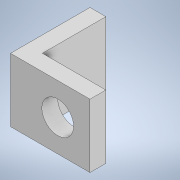
# Autodesk Inventor part: sideSupport
Saved by Autodesk Inventor 2022.2 (Build 262287010, 287A)
## iProperties
Created: 2022-09-12
Part Number: sideSupport
Material: Generic
Document SubType Name: Modeling
Designer: robst
Density: 1 g/cm^3
Appearance: Default
Author: robst
Autodesk Inventor part; units mm, degrees
ref_plane "YZ Plane" through (0, 0, 0) normal (1, 0, 0) x (0, 1, 0)
ref_plane "XZ Plane" through (0, 0, 0) normal (0, 1, 0) x (-1, 0, 0)
ref_plane "XY Plane" through (0, 0, 0) normal (0, 0, 1) x (1, 0, 0)
sketch "Sketch1" plane through (0, 0, 0) normal (1, 0, 0) x (0, 1, 0)
  line L0 (-12.7, 15.875) -> (-12.7, -15.875)
  line L1 (-12.7, -15.875) -> (12.7, -15.875)
  line L2 (12.7, -15.875) -> (12.7, 15.875)
  line L3 (12.7, 15.875) -> (-12.7, 15.875)
  line L4 (-12.7, 15.875) -> (12.7, -15.875) construction
  line L5 (-12.7, -15.875) -> (12.7, 15.875) construction
  point P0 (0, 0)
  dimension "d0" = 25.4
  dimension "d1" = 31.75
  constraints: 12 end point, 2 midpoint, 2 parallel, 1 perpendicular, 1 vertical
  measures "d0" distance of L0.end L1.end
  measures "d1" distance of L1.end L2.end
extrude "Extrusion1" add sketch "Sketch1" against normal blind 6.35
sketch "Sketch2" plane through (0, 0, 0) normal (1, 0, 0) x (0, 0, -1)
  line L0 (-15.875, -12.7) -> (-15.875, 12.7) projected
  line L1 (15.875, -12.7) -> (-15.875, -12.7) projected
  line L2 (-15.875, 12.7) -> (-9.525, 12.7)
  line L3 (-9.525, 12.7) -> (-9.525, -12.7)
  line L4 (-9.525, -12.7) -> (-15.875, -12.7)
  line L5 (-15.875, -12.7) -> (-15.875, 12.7)
  point P0 (0, 0)
  dimension "d4" = 6.35
  constraints: 8 end point, 2 parallel, 1 horizontal, 1 perpendicular, 1 point on line
  measures "d4" distance of L0.end L2.end
extrude "Extrusion2" add sketch "Sketch2" along normal blind 25.4
sketch "Sketch3" plane through (-6.35, -12.7, 15.875) normal (0, 0, 1) x (1, 0, 0)
  circle A0 centre (18.8501, 12.7) radius 6.35
  line L0 (0, 0) -> (0, 25.4) projected
  point P0 (6.35, 12.7)
  dimension "d7" = 18.8501
  dimension "d8" = 12.7
  constraints: 1 centre point
  measures "d7" distance from line of A0.centre L0
  measures "d8" diameter of A0
extrude "Extrusion3" cut sketch "Sketch3" against normal through all
body "Solid1"
